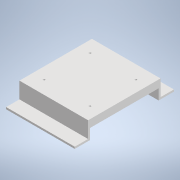
# Autodesk Inventor part: TurntableBase
Saved by Autodesk Inventor 2020 (Build 240168000, 168)
## iProperties
Created: 2022-01-15
Part Number: TurntableBase
Material: Generic
Document SubType Name: Modeling
Designer: danie
Density: 1 g/cm^3
Appearance: Default
Author: danie
Autodesk Inventor part; units mm, degrees
ref_plane "YZ Plane" through (0, 0, 0) normal (1, 0, 0) x (0, 1, 0)
ref_plane "XZ Plane" through (0, 0, 0) normal (0, 1, 0) x (-1, 0, 0)
ref_plane "XY Plane" through (0, 0, 0) normal (0, 0, 1) x (1, 0, 0)
sketch "Sketch1" plane through (0, 0, 0) normal (0, 1, 0) x (-1, 0, 0)
  line L0 (0, 0) -> (-114.3, 0)
  line L1 (-114.3, 0) -> (-114.3, -114.3)
  line L2 (-114.3, -114.3) -> (0, -114.3)
  line L3 (0, -114.3) -> (0, 0)
  dimension "d0" = 114.3
  dimension "d1" = 114.3
  constraints: 8 end point, 2 parallel, 1 horizontal, 1 perpendicular
  measures "d0" distance of L2.end L1.end
  measures "d1" distance of L1.end L0.end
extrude "Extrusion1" add sketch "Sketch1" along normal blind 3.175
sketch "Sketch2" plane through (0, 0, 0) normal (0, 0, 1) x (1, 0, 0)
  line L0 (114.3, 3.175) -> (0, 3.175) projected
  line L1 (0, 3.175) -> (114.3, 3.175)
  line L2 (0, 0) -> (0, 3.175) projected
  line L3 (0, 3.175) -> (114.3, 3.175)
  line L4 (114.3, 3.175) -> (114.3, -26.9875)
  line L5 (114.3, -26.9875) -> (0, -26.9875)
  line L6 (0, -26.9875) -> (0, 3.175)
  dimension "d14" = 30.1625
  constraints: 10 end point, 2 horizontal, 2 parallel, 1 perpendicular
  measures "d14" distance of L3.end L4.end
extrude "Extrusion2" add sketch "Sketch2" along normal blind 3.175
sketch "Sketch5" plane through (114.3, 0, -114.3) normal (0, 0, -1) x (-1, 0, 0)
  line L0 (114.3, 3.175) -> (114.3, -26.9875) projected
  line L1 (0, 3.175) -> (114.3, 3.175)
  line L2 (114.3, 3.175) -> (114.3, -26.9875)
  line L3 (114.3, -26.9875) -> (0, -26.9875)
  line L4 (0, -26.9875) -> (0, 3.175)
  point P0 (114.3, 0)
  constraints: 8 end point, 2 parallel, 1 horizontal, 1 perpendicular
extrude "Extrusion5" add sketch "Sketch5" along normal blind 3.175
sketch "Sketch6" plane through (0, -26.9875, -114.3) normal (0, -1, 0) x (1, 0, 0)
  line L0 (114.3, 114.3) -> (114.3, 0) projected
  line L1 (114.3, 0) -> (0, 0)
  line L2 (0, 0) -> (0, -25.4)
  line L3 (0, -25.4) -> (114.3, -25.4)
  line L4 (114.3, -25.4) -> (114.3, 0)
  line L5 (0, 114.3) -> (114.3, 114.3) projected
  line L6 (114.3, 114.3) -> (0, 114.3)
  line L7 (0, 114.3) -> (0, 139.7)
  line L8 (0, 139.7) -> (114.3, 139.7)
  line L9 (114.3, 139.7) -> (114.3, 114.3)
  dimension "d17" = 25.4
  dimension "d18" = 25.4
  constraints: 16 end point, 4 parallel, 2 horizontal, 2 perpendicular, 1 point on line
  measures "d17" distance of L2.end L1.end
  measures "d18" distance of L6.end L7.end
extrude "Extrusion6" add sketch "Sketch6" against normal blind 3.175
sketch "Sketch7" plane through (0, -23.8125, -114.3) normal (0, 1, 0) x (1, 0, 0)
  point P0 (0, -114.3)
sketch "Sketch8" plane through (0, 3.175, 0) normal (0, 1, 0) x (1, 0, 0)
  circle A0 centre (19.0626, 18.7934) radius 1.5875
  circle A1 centre (19.0626, 95.3281) radius 1.5875
  circle A2 centre (95.4804, 18.7934) radius 1.5875
  circle A3 centre (95.4804, 95.3281) radius 1.5875
  point P0 (0, 0)
  dimension "d21" = 3.175
  dimension "d22" = 3.175
  dimension "d23" = 3.175
  dimension "d24" = 3.175
  constraints: 4 centre point
  measures "d21" diameter of A0
  measures "d22" diameter of A1
  measures "d23" diameter of A2
  measures "d24" diameter of A3
extrude "Extrusion7" cut sketch "Sketch8" against normal blind 12.7
sketch "Sketch9" plane through (0, -23.8125, -114.3) normal (0, 1, 0) x (1, 0, 0)
  line L0 (114.3, -139.7) -> (0, -139.7) construction
  line L1 (0, -139.7) -> (0, -127) construction
  line L2 (0, -114.3) -> (0, -139.7) construction
  line L3 (0, -139.7) -> (12.7, -139.7) construction
  line L4 (114.3, -114.3) -> (114.3, -139.7) construction
  line L5 (0, -127) -> (28.575, -127) construction
  line L6 (0, -127) -> (28.575, -127) construction
  line L7 (28.575, -127) -> (85.725, -127) construction
  circle A0 centre (28.575, -127) radius 3.175
  circle A1 centre (85.725, -127) radius 3.175
  line L8 (114.3, 25.4) -> (0, 25.4) construction
  line L9 (0, 25.4) -> (0, 12.7) construction
  line L10 (0, 12.7) -> (28.575, 12.7) construction
  line L11 (28.575, 12.7) -> (85.725, 12.7) construction
  line L12 (28.575, 12.7) -> (85.725, 12.7) construction
  circle A2 centre (28.575, 12.7) radius 3.175
  circle A3 centre (85.725, 12.7) radius 3.175
  dimension "d27" = 12.7
  dimension "d28" = 90
  dimension "d29" = 28.575
  dimension "d30" = 0
  dimension "d31" = 57.15
  dimension "d33" = 6.35
  dimension "d34" = 6.35
  dimension "d35" = 12.7
  dimension "d36" = 28.575
  dimension "d37" = 57.15
  dimension "d39" = 6.35
  dimension "d40" = 6.35
  constraints: 18 end point, 5 horizontal, 4 centre point, 4 coincident, 3 equal length, 1 collinear, 1 perpendicular, 1 vertical
  measures "d27" distance of L0.end L1.end
  measures "d28" angle of L3 L1
  measures "d29" distance of L1.end L5.end
  measures "d30" distance between parallel lines of L5 L6
  measures "d31" distance of L6.end L7.end
  measures "d33" diameter of A0
  measures "d34" diameter of A1
  measures "d35" distance of L8.end L9.end
  measures "d36" distance of L9.end L10.end
  measures "d37" distance of L10.end L11.end
  measures "d39" diameter of A2
  measures "d40" diameter of A3
extrude "Extrusion8" cut sketch "Sketch9" against normal blind 3.175
sketch "Sketch10" plane through (0, 0, 0) normal (0, -1, 0) x (1, 0, 0)
  line L0 (0, 0) -> (114.3, 0) projected
  line L1 (114.3, -117.475) -> (0, -117.475) projected
  line L2 (114.3, 0) -> (0, 0)
  line L3 (0, 0) -> (0, -117.475)
  line L4 (0, -117.475) -> (114.3, -117.475)
  line L5 (114.3, -117.475) -> (114.3, 0)
  circle A0 centre (95.4804, -18.7934) radius 1.5875 projected
  circle A1 centre (95.4804, -18.7934) radius 1.5875
  circle A2 centre (95.4804, -95.3281) radius 1.5875 projected
  circle A3 centre (95.4804, -95.3281) radius 1.5875
  circle A4 centre (19.0626, -18.7934) radius 1.5875 projected
  circle A5 centre (19.0626, -18.7934) radius 1.5875
  circle A6 centre (19.0626, -95.3281) radius 1.5875 projected
  circle A7 centre (19.0626, -95.3281) radius 1.5875
  dimension "d45" = 3.175
  dimension "d46" = 3.175
  dimension "d47" = 3.175
  dimension "d48" = 3.175
  constraints: 8 end point, 4 centre point, 4 coincident, 2 parallel, 1 horizontal, 1 perpendicular
  measures "d45" diameter of A1
  measures "d46" diameter of A3
  measures "d47" diameter of A5
  measures "d48" diameter of A7
extrude "Extrusion9" add sketch "Sketch10" along normal blind 9.525
body "Solid1"
